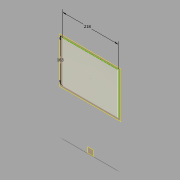
# Autodesk Inventor part: midwall-0
Saved by Autodesk Inventor 2022 (Build 260153000, 153)
## iProperties
Created: 2021-12-10
Part Number: midwall-0
Material: Серебро
Document SubType Name: Modeling
Designer: kalugin_a
Mass: 111.74 g
Surface Area: 819.236 cm^2
Volume: 558.7 cm^3
Density: 10.49 g/cm^3
Appearance: Гладкий — слоновая кость
Author: kalugin_a
Autodesk Inventor part; units mm, degrees
ref_plane "YZ Plane" through (0, 0, 0) normal (1, 0, 0) x (0, 1, 0)
ref_plane "XZ Plane" through (0, 0, 0) normal (0, 1, 0) x (-1, 0, 0)
ref_plane "XY Plane" through (0, 0, 0) normal (0, 0, 1) x (1, 0, 0)
ref_plane "РабПлоскость5" through (0.2962, -249.01, 34.8743) normal (0, 0, 1) x (1, 0, 0)
sketch "Эскиз1" plane through (0.2962, -249.01, 34.8743) normal (0, 0, 1) x (1, 0, 0)
  line L0 (-109.7667, 333.6792) -> (108.2333, 333.6792)
  line L1 (108.2333, 333.6792) -> (108.2333, 170.6792)
  line L2 (108.2333, 170.6792) -> (-109.7667, 170.6792)
  line L3 (-109.7667, 170.6792) -> (-109.7667, 333.6792)
  point P0 (-0.2962, 249.01)
  dimension "d2" = 218
  dimension "d3" = 163
  constraints: 8 end point, 2 parallel, 1 horizontal, 1 perpendicular
  measures "d2" distance of L0.start L0.end
  measures "d3" distance between parallel lines of L2 L0
extrude "Выдавливание1" add sketch "Эскиз1" along normal blind 2
ref_plane "РабПлоскость6" through (0.2962, -249.01, 35.8743) normal (0, 0, 1) x (1, 0, 0)
